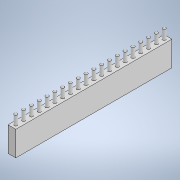
# Autodesk Inventor part: Гребенка 20 МАМА
Saved by Autodesk Inventor 2020 (Build 240168000, 168)
## iProperties
Created: 2021-08-09
Part Number: Гребенка 20 МАМА
Material: Типовые
Document SubType Name: Modeling
Designer: Антон
Density: 1 g/cm^3
Appearance: По умолчанию
Author: Антон
Autodesk Inventor part; units mm, degrees
ref_plane "YZ Plane" through (0, 0, 0) normal (1, 0, 0) x (0, 1, 0)
ref_plane "XZ Plane" through (0, 0, 0) normal (0, 1, 0) x (-1, 0, 0)
ref_plane "XY Plane" through (0, 0, 0) normal (0, 0, 1) x (1, 0, 0)
sketch "Эскиз1" plane through (0, 0, 0) normal (0, 1, 0) x (-1, 0, 0)
  line L0 (0, 0) -> (2.52, 0)
  line L1 (2.52, 0) -> (2.52, -2.52)
  line L2 (2.52, -2.52) -> (0, -2.52)
  line L3 (0, -2.52) -> (0, 0)
  dimension "d1" = 2.52
  dimension "d2" = 2.52
  constraints: 8 end point, 2 parallel, 1 horizontal, 1 perpendicular
  measures "d1" distance of L1.end L2.end
  measures "d2" distance of L0.end L1.end
extrude "Выдавливание1" add sketch "Эскиз1" along normal blind 8
sketch "Эскиз2" plane through (0, 8, 0) normal (0, 1, 0) x (1, 0, 0)
  line L0 (-2.52, 2.52) -> (-2.52, 0) construction
  line L1 (0, 0) -> (0, 2.52) construction
  line L2 (-2.52, 0) -> (0, 2.52) construction
  circle A0 centre (-1.26, 1.26) radius 0.5
  dimension "d22" = 1
  constraints: 2 end point, 1 centre point, 1 midpoint
  measures "d22" diameter of A0
extrude "Выдавливание2" add sketch "Эскиз2" along normal blind 3.5
chamfer "Фаска3" distance 0.5 angle 45 1 edges at (-1.76, 11.5, -1.26)
sketch "Эскиз3" plane through (0, 0, 0) normal (0, -1, 0) x (1, 0, 0)
  line L0 (0, 0) -> (0, -2.52) construction
  line L1 (0, -2.52) -> (-2.52, -2.52) construction
  line L2 (0, 0) -> (-2.52, -2.52) construction
  line L3 (-1.81, -0.71) -> (-0.71, -0.71)
  line L4 (-0.71, -0.71) -> (-0.71, -1.81)
  line L5 (-0.71, -1.81) -> (-1.81, -1.81)
  line L6 (-1.81, -1.81) -> (-1.81, -0.71)
  line L7 (-1.81, -0.71) -> (-0.71, -1.81) construction
  line L8 (-0.71, -0.71) -> (-1.81, -1.81) construction
  point P0 (-1.26, -1.26)
  dimension "d15" = 1.1
  dimension "d16" = 1.1
  constraints: 14 end point, 2 midpoint, 2 parallel, 1 horizontal, 1 perpendicular
  measures "d15" distance of L4.end L5.end
  measures "d16" distance of L3.end L4.end
extrude "Выдавливание3" cut sketch "Эскиз3" against normal blind 6
pattern_linear "Прямоуг.массив1" count 20 spacing 2.52 along (0, 0, 1) of "Выдавливание1", "Выдавливание2", "Выдавливание3", "Фаска3"
